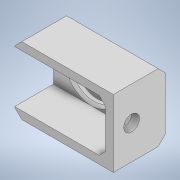
# Autodesk Inventor part: LED_Holder_Button_Holder
Saved by Autodesk Inventor 2021 (Build 250183000, 183)
## iProperties
Created: 2021-02-24
Part Number: LED_Holder_Button_Holder
Material: Generic
Document SubType Name: Modeling
Designer: Viktor
Density: 1 g/cm^3
Appearance: Default
Author: Viktor
## iProperties of the stored document _3DPrint.ipt
Created: 2021-02-24
Part Number: _3DPrint
Material: Generic
Document SubType Name: Modeling
Designer: Viktor
Density: 1 g/cm^3
Appearance: Default
Author: Viktor
Autodesk Inventor part; units mm, degrees
ref_plane "YZ Plane" through (0, 0, 0) normal (1, 0, 0) x (0, 1, 0)
ref_plane "XZ Plane" through (0, 0, 0) normal (0, 1, 0) x (-1, 0, 0)
ref_plane "XY Plane" through (0, 0, 0) normal (0, 0, 1) x (1, 0, 0)
sketch "Sketch1" plane through (0, 0, 0) normal (0, 0, 1) x (1, 0, 0)
  line L0 (-19, -13) -> (19, -13)
  line L1 (19, -13) -> (19, 13)
  line L2 (19, 13) -> (-19, 13)
  line L3 (-19, 13) -> (-19, -13)
  line L4 (-19, -13) -> (19, 13) construction
  line L5 (19, -13) -> (-19, 13) construction
  point P0 (0, 0)
  dimension "d0" = 26
  dimension "d1" = 38
  constraints: 12 end point, 2 midpoint, 2 parallel, 1 horizontal, 1 perpendicular
  measures "d0" distance between parallel lines of L0 L2
  measures "d1" distance between parallel lines of L1 L3
extrude "Extrusion1" add sketch "Sketch1" along normal blind 20
sketch "Sketch2" plane through (0, 0, 20) normal (0, 0, 1) x (1, 0, 0)
  line L0 (-26.6, 0) -> (26.6, 0) projected
  line L1 (-19, 10) -> (10, 10)
  line L2 (10, 10) -> (10, -10)
  line L3 (10, -10) -> (-19, -10)
  line L4 (-19, -10) -> (-19, 10)
  line L5 (-19, 10) -> (10, -10) construction
  line L6 (10, 10) -> (-19, -10) construction
  line L7 (19, 13) -> (-19, 13) projected
  line L8 (19, -13) -> (19, 13) projected
  line L9 (-19, 13) -> (-19, -13) projected
  line L10 (10, 10) -> (16, 10)
  line L11 (16, 10) -> (16, -10)
  line L12 (16, -10) -> (10, -10)
  line L13 (10, -10) -> (10, 10)
  point P0 (0, 0)
  point P1 (-4.5, 0)
  point P2 (-19, 0)
  dimension "d5" = 20
  dimension "d7" = 29
  dimension "d8" = 9
  dimension "d9" = 3
  constraints: 20 end point, 4 midpoint, 4 parallel, 2 horizontal, 2 perpendicular, 2 point on line
  measures "d5" distance between parallel lines of L3 L1
  measures "d7" distance between parallel lines of L4 L2
  measures "d8" distance between parallel lines of L2 L8
  measures "d9" distance between parallel lines of L8 L11
extrude "Extrusion2" cut sketch "Sketch2" against normal blind 15 contours L4 L1 L2 L0 | L0 L2 L3 L4 | L2 L10 L11 L0 | L0 L11 L12 L2
sketch "Sketch3" plane through (0, 0, 5) normal (0, 0, 1) x (1, 0, 0)
  line L0 (-26.6, 0) -> (26.6, 0) projected
  circle A0 centre (-4.5, 0) radius 9
  line L1 (-19, -10) -> (-19, 10) projected
  point P0 (0, 0)
  dimension "d12" = 18
  dimension "d13" = 14.5
  constraints: 1 centre point, 1 point on line
  measures "d12" diameter of A0
  measures "d13" distance from line of L1 A0.centre
extrude "Extrusion3" cut sketch "Sketch3" against normal blind 2.5
sketch "Sketch4" plane through (-4.5, 0, 2.5) normal (0, 0, 1) x (1, 0, 0)
  circle A0 centre (0, 0) radius 9 projected
  circle A1 centre (0, 0) radius 6.25
  point P0 (4.5, 0)
  dimension "d16" = 12.5
  constraints: 1 centre point, 1 coincident
  measures "d16" diameter of A1
extrude "Extrusion4" cut sketch "Sketch4" against normal blind 2.5 contours A1
chamfer "Chamfer1" distance 1 angle 45 1 edges at (-13.5, 0, 5)
chamfer "Chamfer2" distance 1 angle 45 1 edges at (-10.75, 0, 2.5)
chamfer "Chamfer3" distance 2.5 angle 45 2 edges at (16, -10, 12.5) (16, 10, 12.5)
chamfer "Chamfer5" distance 1 angle 45 1 edges at (16, 0, 5)
sketch "Sketch5" plane through (16, -7.5, 20) normal (-1, 0, 0) x (0, 0, 1)
  line L0 (-24, 7.5) -> (4, 7.5) projected
  circle A0 centre (-7, 7.5) radius 3
  line L1 (0, 15) -> (0, 0) projected
  point P0 (-20, 7.5)
  dimension "d34" = 6
  dimension "d35" = 7
  constraints: 1 centre point, 1 point on line
  measures "d34" diameter of A0
  measures "d35" distance from line of L1 A0.centre
extrude "Extrusion5" cut sketch "Sketch5" against normal through all
chamfer "Chamfer6" distance 2.75 angle 45 5 edges at (0, -13, 0) (-19, 0, 0) (0, 13, 0) (-19, 13, 10) (-19, -13, 10)
body "Solid1"
